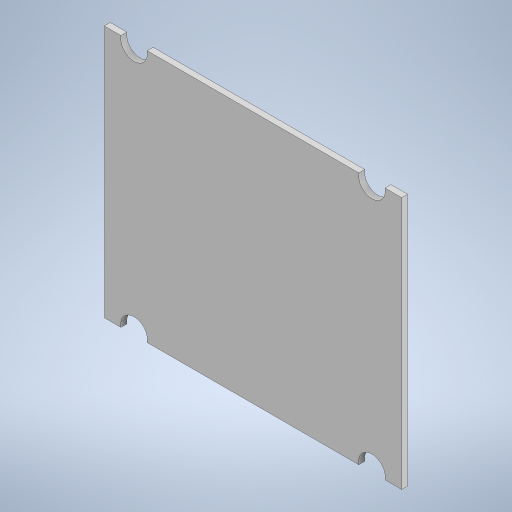
# Autodesk Inventor part: 카메라
Saved by Autodesk Inventor 2023 (Build 270158000, 158)
## iProperties
Created: 2022-11-10
Part Number: 카메라
Material: 일반
Document SubType Name: Modeling
Designer: user
Density: 1 g/cm^3
Appearance: 기본값
Author: user
Autodesk Inventor part; units mm, degrees
ref_plane "YZ Plane" through (0, 0, 0) normal (1, 0, 0) x (0, 1, 0)
ref_plane "XZ Plane" through (0, 0, 0) normal (0, 1, 0) x (-1, 0, 0)
ref_plane "XY Plane" through (0, 0, 0) normal (0, 0, 1) x (1, 0, 0)
sketch "스케치1" plane through (0, 0, 0) normal (0, 0, 1) x (1, 0, 0)
  line L0 (-15, 12.75) -> (15, 12.75)
  line L1 (15, 12.75) -> (15, -12.75)
  line L2 (15, -12.75) -> (-15, -12.75)
  line L3 (-15, -12.75) -> (-15, 12.75)
  line L4 (-15, 12.75) -> (15, -12.75) construction
  line L5 (15, 12.75) -> (-15, -12.75) construction
  point P0 (0, 0)
  dimension "d0" = 30
  dimension "d1" = 25.5
  constraints: 12 end point, 2 midpoint, 2 parallel, 1 horizontal, 1 perpendicular
  measures "d0" distance of L1.end L2.end
  measures "d1" distance of L0.end L1.end
extrude "돌출1" add sketch "스케치1" along normal blind 0.6
sketch "스케치2" plane through (0, 0, 0.6) normal (0, 0, 1) x (1, 0, 0)
  line L0 (-12, 12.5) -> (12, 12.5) construction
  line L1 (12, 12.5) -> (12, -12.5) construction
  line L2 (12, -12.5) -> (-12, -12.5) construction
  line L3 (-12, -12.5) -> (-12, 12.5) construction
  line L4 (-12, 12.5) -> (12, -12.5) construction
  line L5 (12, 12.5) -> (-12, -12.5) construction
  circle A0 centre (-12, 12.5) radius 1.35
  line L6 (0, 0) -> (2.9339, 0)
  line L7 (0, 0) -> (0, 3.0969)
  circle A1 centre (12, 12.5) radius 1.35
  circle A2 centre (-12, -12.5) radius 1.35
  circle A3 centre (12, -12.5) radius 1.35
  dimension "d4" = 24
  dimension "d5" = 25
  dimension "d6" = 2.7
  constraints: 16 end point, 4 centre point, 3 symmetric about line, 2 horizontal, 2 midpoint, 2 parallel, 1 coincident, 1 perpendicular, 1 vertical, 3 other
  measures "d4" distance of L1.end L2.end
  measures "d5" distance of L0.end L1.end
  measures "d6" diameter of A0
extrude "돌출2" cut sketch "스케치2" against normal blind 0.6
